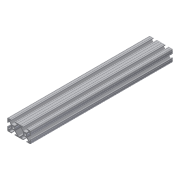
# Autodesk Inventor part: 1020 Extrusion x 12in
Saved by Autodesk Inventor 2013 (Build 170138000, 138)
## iProperties
Created: 2014-02-05
Part Number: 1020 Extrusion x 12in
Material: Aluminum 6061
Document SubType Name: Modeling
Designer: Nemo
Density: 1 g/cm^3
Author: Nemo
Autodesk Inventor part; units mm, degrees
ref_plane "YZ Plane" through (0, 0, 0) normal (1, 0, 0) x (0, 1, 0)
ref_plane "XZ Plane" through (0, 0, 0) normal (0, 1, 0) x (-1, 0, 0)
ref_plane "XY Plane" through (0, 0, 0) normal (0, 0, 1) x (1, 0, 0)
sketch "1020 profile" plane through (0, 0, 0) normal (0, 0, 1) x (1, 0, 0)
  line L0 (-16.9828, 23.1902) -> (-14.8539, 23.1902)
  arc A0 (-16.8995, 25.4) -> (-15.8835, 25.4) centre (-16.3915, 25.4) ccw
  line L1 (-14.8538, 25.4) -> (-15.8835, 25.4)
  arc A1 (-14.8539, 23.1902) -> (-13.8049, 24.2392) centre (-14.8539, 24.2392) ccw
  arc A2 (-13.8049, 24.351) -> (-14.8538, 25.4) centre (-14.8538, 24.351) ccw
  line L2 (-13.8049, 24.2392) -> (-13.8049, 24.351)
  arc A3 (-16.9828, 23.1902) -> (-17.7338, 21.3661) centre (-16.9828, 22.1235) ccw
  line L3 (-14.4564, 18.1163) -> (-17.7338, 21.3661)
  line L4 (-16.8995, 25.4) -> (-20.1168, 25.4)
  arc A4 (-21.1328, 25.3998) -> (-20.1168, 25.4) centre (-20.6248, 25.4) ccw
  arc A5 (-21.1328, 25.3998) -> (-23.2662, 23.2664) centre (-21.1582, 23.2918) ccw
  line L5 (-19.3004, 19.7665) -> (-16.0143, 16.5082)
  arc A6 (-19.3004, 19.7665) -> (-21.0566, 19.0347) centre (-20.026, 19.0347) ccw
  arc A7 (-23.2664, 22.2504) -> (-23.2662, 23.2664) centre (-23.2664, 22.7584) ccw
  line L6 (-23.2664, 22.2504) -> (-23.2664, 19.0331)
  arc A8 (-23.2664, 18.0171) -> (-23.2664, 19.0331) centre (-23.2664, 18.5251) ccw
  line L7 (-23.2664, 18.0171) -> (-23.2664, 16.9375)
  line L8 (-21.0566, 16.9875) -> (-21.0566, 19.0347)
  arc A9 (-23.2664, 16.9375) -> (-22.2674, 15.9385) centre (-22.2674, 16.9375) ccw
  line L9 (-22.2674, 15.9385) -> (-22.1056, 15.9385)
  line L10 (-22.1056, 9.4615) -> (-22.2174, 9.4615)
  arc A10 (-21.0566, 8.4125) -> (-22.1056, 9.4615) centre (-22.1056, 8.4125) ccw
  arc A11 (-16.0069, 8.7577) -> (-15.0749, 11.0048) centre (-18.2499, 11.0048) ccw
  arc A12 (-22.2174, 9.4615) -> (-23.2664, 8.4125) centre (-22.2174, 8.4125) ccw
  arc A13 (2.5668, 2.667) -> (3.6794, 3.1272) centre (2.5668, 4.2418) ccw
  line L11 (1.7004, 2.667) -> (2.5668, 2.667)
  arc A14 (0.5879, 3.1272) -> (1.7004, 2.667) centre (1.7004, 4.2418) ccw
  line L12 (0, 0) -> (4.2672, 0)
  line L13 (21.25, 2.2098) -> (19.1211, 2.2098)
  arc A15 (21.1667, 0) -> (20.1507, 0) centre (20.6587, 0) ccw
  line L14 (19.1211, 0) -> (20.1507, 0)
  arc A16 (19.1211, 2.2098) -> (18.0721, 1.1608) centre (19.1211, 1.1608) ccw
  arc A17 (18.0721, 1.049) -> (19.1211, 0) centre (19.1211, 1.049) ccw
  line L15 (18.0721, 1.1608) -> (18.0721, 1.049)
  arc A18 (20.243, 16.5465) -> (19.3421, 14.3308) centre (22.5171, 14.3308) ccw
  arc A19 (16.4785, 17.1958) -> (18.7526, 18.1551) centre (16.4785, 20.3708) ccw
  arc A20 (19.3421, 11.0692) -> (20.4318, 8.675) centre (22.5171, 11.0692) ccw
  line L16 (16.4785, 17.1958) -> (13.2169, 17.1958)
  arc A21 (10.9506, 18.1472) -> (13.2169, 17.1958) centre (13.2169, 20.3708) ccw
  arc A22 (18.3215, 7.4234) -> (16.2362, 8.2042) centre (16.2362, 5.0292) ccw
  circle A23 centre (14.8336, 12.7) radius 2.6035
  line L17 (12.9746, 8.2042) -> (16.2362, 8.2042)
  arc A24 (12.9746, 8.2042) -> (10.7315, 7.2763) centre (12.9746, 5.0292) ccw
  line L18 (19.3421, 11.0692) -> (19.3421, 14.3308)
  line L19 (10.3251, 11.0777) -> (10.3251, 14.3223)
  arc A25 (10.3251, 14.3223) -> (9.4165, 16.5459) centre (7.1501, 14.3223) ccw
  line L20 (9.4165, 16.5459) -> (3.8092, 22.2611)
  line L21 (10.9506, 18.1472) -> (7.6978, 21.4627)
  line L22 (19.1211, 23.1902) -> (21.25, 23.1902)
  arc A26 (18.0721, 24.2392) -> (19.1211, 23.1902) centre (19.1211, 24.2392) ccw
  line L23 (18.0721, 24.351) -> (18.0721, 24.2392)
  line L24 (20.1507, 25.4) -> (19.1211, 25.4)
  arc A27 (19.1211, 25.4) -> (18.0721, 24.351) centre (19.1211, 24.351) ccw
  arc A28 (20.1507, 25.4) -> (21.1667, 25.4) centre (20.6587, 25.4) ccw
  arc A29 (-3.399, 21.3661) -> (-4.15, 23.1902) centre (-4.15, 22.1235) ccw
  line L25 (-1.016, 25.4) -> (-4.2333, 25.4)
  arc A30 (-5.2493, 25.4) -> (-4.2333, 25.4) centre (-4.7413, 25.4) ccw
  line L26 (0.6296, 22.2765) -> (-5.1184, 16.5768)
  line L27 (-6.2789, 23.1902) -> (-4.15, 23.1902)
  line L28 (-5.2493, 25.4) -> (-6.2789, 25.4)
  line L29 (-3.399, 21.3661) -> (-6.6764, 18.1163)
  arc A31 (-7.3279, 24.2392) -> (-6.2789, 23.1902) centre (-6.2789, 24.2392) ccw
  line L30 (-7.3279, 24.351) -> (-7.3279, 24.2392)
  arc A32 (-6.2789, 25.4) -> (-7.3279, 24.351) centre (-6.2789, 24.351) ccw
  arc A33 (-1.016, 25.4) -> (0, 25.4) centre (-0.508, 25.4) ccw
  arc A34 (-5.1184, 16.5768) -> (-6.0579, 14.3223) centre (-2.8829, 14.3223) ccw
  line L31 (-6.0579, 14.3223) -> (-6.0579, 11.0777)
  arc A35 (-6.0579, 11.0777) -> (-5.1259, 8.8306) centre (-2.8829, 11.0777) ccw
  arc A36 (-8.9119, 17.1958) -> (-6.6764, 18.1163) centre (-8.9119, 20.3708) ccw
  line L32 (-8.9119, 17.1958) -> (-12.2209, 17.1958)
  arc A37 (-14.4564, 18.1163) -> (-12.2209, 17.1958) centre (-12.2209, 20.3708) ccw
  arc A38 (-15.0749, 14.2536) -> (-16.0143, 16.5082) centre (-18.2499, 14.2536) ccw
  line L33 (-15.0749, 14.2536) -> (-15.0749, 11.0048)
  circle A39 centre (-10.5664, 12.7) radius 2.6035
  line L34 (-12.12, 8.2042) -> (-9.0128, 8.2042)
  arc A40 (-12.12, 8.2042) -> (-14.363, 7.2763) centre (-12.12, 5.0292) ccw
  arc A41 (-22.1056, 15.9385) -> (-21.0566, 16.9875) centre (-22.1056, 16.9875) ccw
  arc A42 (8.423, 23.1902) -> (7.6978, 21.4627) centre (8.423, 22.1742) ccw
  line L35 (8.423, 23.1902) -> (10.5461, 23.1902)
  arc A43 (1.7384, 22.733) -> (0.6296, 22.2765) centre (1.7384, 21.1582) ccw
  line L36 (4.2672, 25.4) -> (0, 25.4)
  line L37 (2.6851, 22.733) -> (1.7384, 22.733)
  arc A44 (3.8092, 22.2611) -> (2.6851, 22.733) centre (2.6851, 21.1582) ccw
  arc A45 (4.2672, 25.4) -> (5.2832, 25.4) centre (4.7752, 25.4) ccw
  line L38 (8.5005, 25.4) -> (5.2832, 25.4)
  arc A46 (8.5005, 25.4) -> (9.5165, 25.4) centre (9.0085, 25.4) ccw
  line L39 (10.5462, 25.4) -> (9.5165, 25.4)
  arc A47 (11.5951, 24.351) -> (10.5462, 25.4) centre (10.5462, 24.351) ccw
  line L40 (11.5951, 24.2392) -> (11.5951, 24.351)
  arc A48 (10.5461, 23.1902) -> (11.5951, 24.2392) centre (10.5461, 24.2392) ccw
  line L41 (-14.8539, 2.2098) -> (-16.9828, 2.2098)
  arc A49 (-15.8835, 0) -> (-16.8995, 0) centre (-16.3915, 0) ccw
  arc A50 (-13.8048, 1.1608) -> (-14.8539, 2.2098) centre (-14.8539, 1.1608) ccw
  line L42 (-15.8835, 0) -> (-14.8539, 0)
  line L43 (-13.8048, 1.049) -> (-13.8048, 1.1608)
  arc A51 (-14.8539, 0) -> (-13.8048, 1.049) centre (-14.8539, 1.049) ccw
  line L44 (-7.3279, 1.1608) -> (-7.3279, 1.049)
  arc A52 (-6.7698, 7.2763) -> (-9.0128, 8.2042) centre (-9.0128, 5.0292) ccw
  arc A53 (-6.2789, 2.2098) -> (-7.3279, 1.1608) centre (-6.2789, 1.1608) ccw
  arc A54 (-7.3279, 1.049) -> (-6.2789, 0) centre (-6.2789, 1.049) ccw
  line L45 (-6.2789, 0) -> (-5.2493, 0)
  arc A55 (-4.2333, 0) -> (-5.2493, 0) centre (-4.7413, 0) ccw
  arc A56 (-4.15, 2.2098) -> (-3.4323, 3.9449) centre (-4.15, 3.2258) ccw
  line L46 (-6.7698, 7.2763) -> (-3.4323, 3.9449)
  line L47 (-4.2333, 0) -> (-1.016, 0)
  arc A57 (0, 0) -> (-1.016, 0) centre (-0.508, 0) ccw
  line L48 (-5.1259, 8.8306) -> (0.5879, 3.1272)
  line L49 (-4.15, 2.2098) -> (-6.2789, 2.2098)
  arc A58 (5.2832, 0) -> (4.2672, 0) centre (4.7752, 0) ccw
  line L50 (5.2832, 0) -> (8.5005, 0)
  arc A59 (9.5165, 0) -> (8.5005, 0) centre (9.0085, 0) ccw
  line L51 (9.5165, 0) -> (10.5461, 0)
  arc A60 (10.5461, 0) -> (11.5952, 1.049) centre (10.5461, 1.049) ccw
  line L52 (11.5952, 1.049) -> (11.5952, 1.1608)
  arc A61 (11.5952, 1.1608) -> (10.5461, 2.2098) centre (10.5461, 1.1608) ccw
  line L53 (10.5461, 2.2098) -> (8.423, 2.2098)
  line L54 (3.6794, 3.1272) -> (9.3931, 8.8306)
  line L55 (7.6143, 4.1647) -> (10.7315, 7.2763)
  arc A62 (9.3931, 8.8306) -> (10.3251, 11.0777) centre (7.1501, 11.0777) ccw
  arc A63 (7.6143, 4.1647) -> (8.423, 2.2098) centre (8.423, 3.3545) ccw
  arc A64 (26.3228, 9.4615) -> (25.3238, 8.4625) centre (26.3228, 8.4625) ccw
  line L56 (26.5346, 9.4615) -> (26.3228, 9.4615)
  arc A65 (27.5336, 8.4625) -> (26.5346, 9.4615) centre (26.5346, 8.4625) ccw
  line L57 (21.9777, 21.4652) -> (18.7526, 18.1551)
  arc A66 (21.9777, 21.4652) -> (21.25, 23.1902) centre (21.25, 22.1742) ccw
  line L58 (24.384, 25.4) -> (21.1667, 25.4)
  line L59 (20.243, 16.5465) -> (23.66, 20.0534)
  arc A67 (24.384, 25.4) -> (25.4, 25.3998) centre (24.892, 25.4) ccw
  arc A68 (25.3238, 19.3769) -> (23.66, 20.0534) centre (24.3543, 19.3769) ccw
  arc A69 (27.5335, 23.2664) -> (25.4, 25.3998) centre (25.4254, 23.2918) ccw
  arc A70 (27.5335, 23.2664) -> (27.5336, 22.2504) centre (27.5336, 22.7584) ccw
  line L60 (27.5336, 19.0332) -> (27.5336, 22.2504)
  line L61 (25.3238, 19.3769) -> (25.3238, 16.9375)
  arc A71 (27.5336, 19.0332) -> (27.5336, 18.0171) centre (27.5336, 18.5251) ccw
  arc A72 (25.3238, 16.9375) -> (26.3228, 15.9385) centre (26.3228, 16.9375) ccw
  line L62 (27.5336, 16.9375) -> (27.5336, 18.0171)
  arc A73 (26.5346, 15.9385) -> (27.5336, 16.9375) centre (26.5346, 16.9375) ccw
  line L63 (26.3228, 15.9385) -> (26.5346, 15.9385)
  line L64 (-23.2664, 8.4125) -> (-23.2664, 7.3829)
  line L65 (-21.0566, 6.202) -> (-21.0566, 8.4125)
  line L66 (-16.0069, 8.7577) -> (-19.298, 5.4726)
  arc A74 (-23.2664, 6.3669) -> (-23.2664, 7.3829) centre (-23.2664, 6.8749) ccw
  line L67 (-17.7005, 3.9449) -> (-14.363, 7.2763)
  arc A75 (-21.0566, 6.202) -> (-19.298, 5.4726) centre (-20.026, 6.202) ccw
  line L68 (-23.2664, 6.3669) -> (-23.2664, 3.1496)
  arc A76 (-23.2662, 2.1336) -> (-23.2664, 3.1496) centre (-23.2664, 2.6416) ccw
  arc A77 (-17.7005, 3.9449) -> (-16.9828, 2.2098) centre (-16.9828, 3.2258) ccw
  arc A78 (-23.2662, 2.1336) -> (-21.1328, 0.0002) centre (-21.1582, 2.1082) ccw
  arc A79 (-20.1168, 0) -> (-21.1328, 0.0002) centre (-20.6248, 0) ccw
  line L69 (-20.1168, 0) -> (-16.8995, 0)
  line L70 (18.3215, 7.4234) -> (22.0019, 4.2178)
  arc A80 (21.25, 2.2098) -> (22.0019, 4.2178) centre (21.25, 3.3545) ccw
  line L71 (21.1667, 0) -> (24.384, 0)
  line L72 (23.7176, 5.8131) -> (20.4318, 8.675)
  arc A81 (25.4, 0.0002) -> (24.384, 0) centre (24.892, 0) ccw
  arc A82 (23.7176, 5.8131) -> (25.3238, 6.5441) centre (24.3543, 6.5441) ccw
  arc A83 (25.4, 0.0002) -> (27.5335, 2.1336) centre (25.4254, 2.1082) ccw
  arc A84 (27.5336, 3.1496) -> (27.5335, 2.1336) centre (27.5336, 2.6416) ccw
  line L73 (27.5336, 3.1496) -> (27.5336, 6.3669)
  line L74 (25.3238, 8.4625) -> (25.3238, 6.5441)
  arc A85 (27.5336, 7.3829) -> (27.5336, 6.3669) centre (27.5336, 6.8749) ccw
  line L75 (27.5336, 7.3829) -> (27.5336, 8.4625)
  point P0 (2.1314, 12.704)
  point P1 (2.1336, 12.7)
sketch "Sketch1" plane through (0, 0, 0) normal (0, 0, 1) x (1, 0, 0)
  line L0 (-19.1164, 10.4902) -> (-16.9875, 10.4902)
  arc A0 (-19.0331, 12.7) -> (-18.0171, 12.7) centre (-18.5251, 12.7) ccw
  line L1 (-16.9875, 12.7) -> (-18.0171, 12.7)
  arc A1 (-16.9875, 10.4902) -> (-15.9385, 11.5392) centre (-16.9875, 11.5392) ccw
  arc A2 (-15.9385, 11.651) -> (-16.9875, 12.7) centre (-16.9875, 11.651) ccw
  line L2 (-15.9385, 11.5392) -> (-15.9385, 11.651)
  arc A3 (-19.1164, 10.4902) -> (-19.8674, 8.6661) centre (-19.1164, 9.4235) ccw
  line L3 (-16.59, 5.4163) -> (-19.8674, 8.6661)
  line L4 (-19.0331, 12.7) -> (-22.2504, 12.7)
  arc A4 (-23.2664, 12.6998) -> (-22.2504, 12.7) centre (-22.7584, 12.7) ccw
  arc A5 (-23.2664, 12.6998) -> (-25.3998, 10.5664) centre (-23.2918, 10.5918) ccw
  line L5 (-21.434, 7.0665) -> (-18.148, 3.8082)
  arc A6 (-21.434, 7.0665) -> (-23.1902, 6.3347) centre (-22.1596, 6.3347) ccw
  arc A7 (-25.4, 9.5504) -> (-25.3998, 10.5664) centre (-25.4, 10.0584) ccw
  line L6 (-25.4, 9.5504) -> (-25.4, 6.3331)
  arc A8 (-25.4, 5.3171) -> (-25.4, 6.3331) centre (-25.4, 5.8251) ccw
  line L7 (-25.4, 5.3171) -> (-25.4, 4.2375)
  line L8 (-23.1902, 4.2875) -> (-23.1902, 6.3347)
  arc A9 (-25.4, 4.2375) -> (-24.401, 3.2385) centre (-24.401, 4.2375) ccw
  line L9 (-24.401, 3.2385) -> (-24.2392, 3.2385)
  line L10 (-24.2392, -3.2385) -> (-24.351, -3.2385)
  arc A10 (-23.1902, -4.2875) -> (-24.2392, -3.2385) centre (-24.2392, -4.2875) ccw
  arc A11 (-18.1405, -3.9423) -> (-17.2085, -1.6952) centre (-20.3835, -1.6952) ccw
  arc A12 (-24.351, -3.2385) -> (-25.4, -4.2875) centre (-24.351, -4.2875) ccw
  arc A13 (0.4332, -10.033) -> (1.5457, -9.5728) centre (0.4332, -8.4582) ccw
  line L11 (-0.4332, -10.033) -> (0.4332, -10.033)
  arc A14 (-1.5457, -9.5728) -> (-0.4332, -10.033) centre (-0.4332, -8.4582) ccw
  line L12 (-2.1336, -12.7) -> (2.1336, -12.7)
  line L13 (19.1164, -10.4902) -> (16.9875, -10.4902)
  arc A15 (19.0331, -12.7) -> (18.0171, -12.7) centre (18.5251, -12.7) ccw
  line L14 (16.9875, -12.7) -> (18.0171, -12.7)
  arc A16 (16.9875, -10.4902) -> (15.9384, -11.5392) centre (16.9875, -11.5392) ccw
  arc A17 (15.9384, -11.651) -> (16.9875, -12.7) centre (16.9875, -11.651) ccw
  line L15 (15.9384, -11.5392) -> (15.9384, -11.651)
  arc A18 (18.1094, 3.8465) -> (17.2085, 1.6308) centre (20.3835, 1.6308) ccw
  arc A19 (14.3449, 4.4958) -> (16.619, 5.4551) centre (14.3449, 7.6708) ccw
  arc A20 (17.2085, -1.6308) -> (18.2982, -4.025) centre (20.3835, -1.6308) ccw
  line L16 (14.3449, 4.4958) -> (11.0833, 4.4958)
  arc A21 (8.817, 5.4472) -> (11.0833, 4.4958) centre (11.0833, 7.6708) ccw
  arc A22 (16.1879, -5.2766) -> (14.1026, -4.4958) centre (14.1026, -7.6708) ccw
  circle A23 centre (12.7, 0) radius 2.6035
  line L17 (10.8409, -4.4958) -> (14.1026, -4.4958)
  arc A24 (10.8409, -4.4958) -> (8.5979, -5.4237) centre (10.8409, -7.6708) ccw
  line L18 (17.2085, -1.6308) -> (17.2085, 1.6308)
  line L19 (8.1915, -1.6223) -> (8.1915, 1.6223)
  arc A25 (8.1915, 1.6223) -> (7.2829, 3.8459) centre (5.0165, 1.6223) ccw
  line L20 (7.2829, 3.8459) -> (1.6756, 9.5611)
  line L21 (8.817, 5.4472) -> (5.5642, 8.7627)
  line L22 (16.9875, 10.4902) -> (19.1164, 10.4902)
  arc A26 (15.9385, 11.5392) -> (16.9875, 10.4902) centre (16.9875, 11.5392) ccw
  line L23 (15.9385, 11.651) -> (15.9385, 11.5392)
  line L24 (18.0171, 12.7) -> (16.9875, 12.7)
  arc A27 (16.9875, 12.7) -> (15.9385, 11.651) centre (16.9875, 11.651) ccw
  arc A28 (18.0171, 12.7) -> (19.0331, 12.7) centre (18.5251, 12.7) ccw
  arc A29 (-5.5326, 8.6661) -> (-6.2836, 10.4902) centre (-6.2836, 9.4235) ccw
  line L25 (-3.1496, 12.7) -> (-6.3669, 12.7)
  arc A30 (-7.3829, 12.7) -> (-6.3669, 12.7) centre (-6.8749, 12.7) ccw
  line L26 (-1.504, 9.5765) -> (-7.252, 3.8768)
  line L27 (-8.4125, 10.4902) -> (-6.2836, 10.4902)
  line L28 (-7.3829, 12.7) -> (-8.4125, 12.7)
  line L29 (-5.5326, 8.6661) -> (-8.81, 5.4163)
  arc A31 (-9.4615, 11.5392) -> (-8.4125, 10.4902) centre (-8.4125, 11.5392) ccw
  line L30 (-9.4615, 11.651) -> (-9.4615, 11.5392)
  arc A32 (-8.4125, 12.7) -> (-9.4615, 11.651) centre (-8.4125, 11.651) ccw
  arc A33 (-3.1496, 12.7) -> (-2.1336, 12.7) centre (-2.6416, 12.7) ccw
  arc A34 (-7.252, 3.8768) -> (-8.1915, 1.6223) centre (-5.0165, 1.6223) ccw
  line L31 (-8.1915, 1.6223) -> (-8.1915, -1.6223)
  arc A35 (-8.1915, -1.6223) -> (-7.2595, -3.8694) centre (-5.0165, -1.6223) ccw
  arc A36 (-11.0455, 4.4958) -> (-8.81, 5.4163) centre (-11.0455, 7.6708) ccw
  line L32 (-11.0455, 4.4958) -> (-14.3545, 4.4958)
  arc A37 (-16.59, 5.4163) -> (-14.3545, 4.4958) centre (-14.3545, 7.6708) ccw
  arc A38 (-17.2085, 1.5536) -> (-18.148, 3.8082) centre (-20.3835, 1.5536) ccw
  line L33 (-17.2085, 1.5536) -> (-17.2085, -1.6952)
  circle A39 centre (-12.7, 0) radius 2.6035
  line L34 (-14.2536, -4.4958) -> (-11.1464, -4.4958)
  arc A40 (-14.2536, -4.4958) -> (-16.4966, -5.4237) centre (-14.2536, -7.6708) ccw
  arc A41 (-24.2392, 3.2385) -> (-23.1902, 4.2875) centre (-24.2392, 4.2875) ccw
  arc A42 (6.2894, 10.4902) -> (5.5642, 8.7627) centre (6.2894, 9.4742) ccw
  line L35 (6.2894, 10.4902) -> (8.4125, 10.4902)
  arc A43 (-0.3952, 10.033) -> (-1.504, 9.5765) centre (-0.3952, 8.4582) ccw
  line L36 (2.1336, 12.7) -> (-2.1336, 12.7)
  line L37 (0.5515, 10.033) -> (-0.3952, 10.033)
  arc A44 (1.6756, 9.5611) -> (0.5515, 10.033) centre (0.5515, 8.4582) ccw
  arc A45 (2.1336, 12.7) -> (3.1496, 12.7) centre (2.6416, 12.7) ccw
  line L38 (6.3669, 12.7) -> (3.1496, 12.7)
  arc A46 (6.3669, 12.7) -> (7.3829, 12.7) centre (6.8749, 12.7) ccw
  line L39 (8.4125, 12.7) -> (7.3829, 12.7)
  arc A47 (9.4615, 11.651) -> (8.4125, 12.7) centre (8.4125, 11.651) ccw
  line L40 (9.4615, 11.5392) -> (9.4615, 11.651)
  arc A48 (8.4125, 10.4902) -> (9.4615, 11.5392) centre (8.4125, 11.5392) ccw
  line L41 (-16.9875, -10.4902) -> (-19.1164, -10.4902)
  arc A49 (-18.0171, -12.7) -> (-19.0331, -12.7) centre (-18.5251, -12.7) ccw
  arc A50 (-15.9384, -11.5392) -> (-16.9875, -10.4902) centre (-16.9875, -11.5392) ccw
  line L42 (-18.0171, -12.7) -> (-16.9875, -12.7)
  line L43 (-15.9384, -11.651) -> (-15.9384, -11.5392)
  arc A51 (-16.9875, -12.7) -> (-15.9384, -11.651) centre (-16.9875, -11.651) ccw
  line L44 (-9.4616, -11.5392) -> (-9.4616, -11.651)
  arc A52 (-8.9034, -5.4237) -> (-11.1464, -4.4958) centre (-11.1464, -7.6708) ccw
  arc A53 (-8.4125, -10.4902) -> (-9.4616, -11.5392) centre (-8.4125, -11.5392) ccw
  arc A54 (-9.4616, -11.651) -> (-8.4125, -12.7) centre (-8.4125, -11.651) ccw
  line L45 (-8.4125, -12.7) -> (-7.3829, -12.7)
  arc A55 (-6.3669, -12.7) -> (-7.3829, -12.7) centre (-6.8749, -12.7) ccw
  arc A56 (-6.2836, -10.4902) -> (-5.5659, -8.7551) centre (-6.2836, -9.4742) ccw
  line L46 (-8.9034, -5.4237) -> (-5.5659, -8.7551)
  line L47 (-6.3669, -12.7) -> (-3.1496, -12.7)
  arc A57 (-2.1336, -12.7) -> (-3.1496, -12.7) centre (-2.6416, -12.7) ccw
  line L48 (-7.2595, -3.8694) -> (-1.5457, -9.5728)
  line L49 (-6.2836, -10.4902) -> (-8.4125, -10.4902)
  arc A58 (3.1496, -12.7) -> (2.1336, -12.7) centre (2.6416, -12.7) ccw
  line L50 (3.1496, -12.7) -> (6.3669, -12.7)
  arc A59 (7.3829, -12.7) -> (6.3669, -12.7) centre (6.8749, -12.7) ccw
  line L51 (7.3829, -12.7) -> (8.4125, -12.7)
  arc A60 (8.4125, -12.7) -> (9.4616, -11.651) centre (8.4125, -11.651) ccw
  line L52 (9.4616, -11.651) -> (9.4616, -11.5392)
  arc A61 (9.4616, -11.5392) -> (8.4125, -10.4902) centre (8.4125, -11.5392) ccw
  line L53 (8.4125, -10.4902) -> (6.2894, -10.4902)
  line L54 (1.5457, -9.5728) -> (7.2595, -3.8694)
  line L55 (5.4807, -8.5353) -> (8.5979, -5.4237)
  arc A62 (7.2595, -3.8694) -> (8.1915, -1.6223) centre (5.0165, -1.6223) ccw
  arc A63 (5.4807, -8.5353) -> (6.2894, -10.4902) centre (6.2894, -9.3455) ccw
  arc A64 (24.1892, -3.2385) -> (23.1902, -4.2375) centre (24.1892, -4.2375) ccw
  line L56 (24.401, -3.2385) -> (24.1892, -3.2385)
  arc A65 (25.4, -4.2375) -> (24.401, -3.2385) centre (24.401, -4.2375) ccw
  line L57 (19.8441, 8.7652) -> (16.619, 5.4551)
  arc A66 (19.8441, 8.7652) -> (19.1164, 10.4902) centre (19.1164, 9.4742) ccw
  line L58 (22.2504, 12.7) -> (19.0331, 12.7)
  line L59 (18.1094, 3.8465) -> (21.5263, 7.3534)
  arc A67 (22.2504, 12.7) -> (23.2664, 12.6998) centre (22.7584, 12.7) ccw
  arc A68 (23.1902, 6.6769) -> (21.5263, 7.3534) centre (22.2207, 6.6769) ccw
  arc A69 (25.3998, 10.5664) -> (23.2664, 12.6998) centre (23.2918, 10.5918) ccw
  arc A70 (25.3998, 10.5664) -> (25.4, 9.5504) centre (25.4, 10.0584) ccw
  line L60 (25.4, 6.3332) -> (25.4, 9.5504)
  line L61 (23.1902, 6.6769) -> (23.1902, 4.2375)
  arc A71 (25.4, 6.3332) -> (25.4, 5.3171) centre (25.4, 5.8251) ccw
  arc A72 (23.1902, 4.2375) -> (24.1892, 3.2385) centre (24.1892, 4.2375) ccw
  line L62 (25.4, 4.2375) -> (25.4, 5.3171)
  arc A73 (24.401, 3.2385) -> (25.4, 4.2375) centre (24.401, 4.2375) ccw
  line L63 (24.1892, 3.2385) -> (24.401, 3.2385)
  line L64 (-25.4, -4.2875) -> (-25.4, -5.3171)
  line L65 (-23.1902, -6.498) -> (-23.1902, -4.2875)
  line L66 (-18.1405, -3.9423) -> (-21.4316, -7.2274)
  arc A74 (-25.4, -6.3331) -> (-25.4, -5.3171) centre (-25.4, -5.8251) ccw
  line L67 (-19.8341, -8.7551) -> (-16.4966, -5.4237)
  arc A75 (-23.1902, -6.498) -> (-21.4316, -7.2274) centre (-22.1596, -6.498) ccw
  line L68 (-25.4, -6.3331) -> (-25.4, -9.5504)
  arc A76 (-25.3998, -10.5664) -> (-25.4, -9.5504) centre (-25.4, -10.0584) ccw
  arc A77 (-19.8341, -8.7551) -> (-19.1164, -10.4902) centre (-19.1164, -9.4742) ccw
  arc A78 (-25.3998, -10.5664) -> (-23.2664, -12.6998) centre (-23.2918, -10.5918) ccw
  arc A79 (-22.2504, -12.7) -> (-23.2664, -12.6998) centre (-22.7584, -12.7) ccw
  line L69 (-22.2504, -12.7) -> (-19.0331, -12.7)
  line L70 (16.1879, -5.2766) -> (19.8682, -8.4822)
  arc A80 (19.1164, -10.4902) -> (19.8682, -8.4822) centre (19.1164, -9.3455) ccw
  line L71 (19.0331, -12.7) -> (22.2504, -12.7)
  line L72 (21.584, -6.8869) -> (18.2982, -4.025)
  arc A81 (23.2664, -12.6998) -> (22.2504, -12.7) centre (22.7584, -12.7) ccw
  arc A82 (21.584, -6.8869) -> (23.1902, -6.1559) centre (22.2207, -6.1559) ccw
  arc A83 (23.2664, -12.6998) -> (25.3998, -10.5664) centre (23.2918, -10.5918) ccw
  arc A84 (25.4, -9.5504) -> (25.3998, -10.5664) centre (25.4, -10.0584) ccw
  line L73 (25.4, -9.5504) -> (25.4, -6.3331)
  line L74 (23.1902, -4.2375) -> (23.1902, -6.1559)
  arc A85 (25.4, -5.3171) -> (25.4, -6.3331) centre (25.4, -5.8251) ccw
  line L75 (25.4, -5.3171) -> (25.4, -4.2375)
  point P0 (0, 0)
  constraints: 1 other
extrude "Extrusion1" add sketch "Sketch1" along normal mid plane 304.8
body "Solid1"
